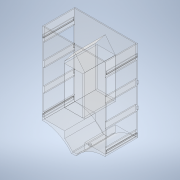
# Autodesk Inventor part: Contenedor
Saved by Autodesk Inventor 2021 (Build 250183000, 183)
## iProperties
Created: 2021-06-28
Part Number: Contenedor
Material: Acrílico, claro
Document SubType Name: Modeling
Designer: artur
Density: 1.19 g/cm^3
Appearance: Transparente - Claro
Mass: 3494.81 g
Surface Area: 8852.35 cm^2
Volume: 2936.81 cm^3
Author: artur
Autodesk Inventor part; units mm, degrees
ref_plane "YZ Plane" through (0, 0, 0) normal (1, 0, 0) x (0, 1, 0)
sketch "Boceto1" plane through (0, 0, 0) normal (0, 0, 1) x (1, 0, 0)
  line L0 (0, 0) -> (100, 0)
  line L1 (0, 300.0017) -> (0, 100.0017)
  line L2 (0, 0) -> (101, 0)
  line L3 (101, 0) -> (101, 400)
  line L4 (101, 400) -> (0, 400)
  line L5 (0, 300.0017) -> (0, 100.0017)
  line L6 (0, 0) -> (98.1777, 0) construction
  line L7 (98.1777, 0) -> (98.1777, 330) construction
  line L8 (98.1777, 330) -> (0, 330) construction
  line L9 (0, 330) -> (0, 0) construction
  line L10 (0, 300.0017) -> (-100, 300.0017) construction
  line L11 (-100, 300.0017) -> (-100, 100.0017) construction
  line L12 (-100, 100.0017) -> (0, 100.0017) construction
  line L13 (0, 100.0017) -> (0, 300.0017) construction
  line L14 (0, 300.0017) -> (-100, 300.0017)
  line L15 (-100, 300.0017) -> (-100, 100.0017)
  line L16 (-100, 100.0017) -> (0, 100.0017)
  line L17 (0, 100.0017) -> (0, 300.0017)
  line L18 (-100, 0) -> (-201, 0)
  line L19 (-201, 0) -> (-201, 400)
  line L20 (-201, 400) -> (-100, 400)
  line L21 (-100, 300.0017) -> (-100, 100.0017)
  line L22 (-100, 0) -> (0, 0)
  line L23 (-100, 400) -> (0, 400)
  line L24 (-95, 105.0017) -> (-5, 105.0017)
  line L25 (-5, 105.0017) -> (-5, 295.0017)
  line L26 (-5, 295.0017) -> (-95, 295.0017)
  line L27 (-95, 295.0017) -> (-95, 105.0017)
  line L28 (106, 400) -> (106, -5)
  line L29 (106, -5) -> (-206, -5)
  line L30 (-206, -5) -> (-206, 400)
  line L31 (-206, 400) -> (-201, 400)
  line L32 (101, 400) -> (106, 400)
  line L33 (-100, 100.0017) -> (-100, 0) construction
  line L34 (-50, -5) -> (-50, -75) construction
  line L35 (-56.35, -74.8888) -> (-43.65, -74.8888)
  line L36 (-43.65, -74.8888) -> (-38.65, -74.8888)
  line L37 (-56.35, -74.8888) -> (-61.35, -74.8888)
  arc A0 (-61.35, -74.8888) -> (-206, -5) centre (-206.1755, -189.9999) ccw
  arc A1 (106, -5) -> (-38.65, -74.8888) centre (106.1755, -189.9999) ccw
  line L38 (-38.65, -74.8888) -> (-38.65, -69.8888)
  line L39 (-61.35, -74.8888) -> (-61.35, -69.8888)
  arc A2 (-61.35, -69.8888) -> (-201, 0) centre (-206.2343, -184.9259) ccw
  arc A3 (98.1777, 0) -> (-38.65, -69.8888) centre (106.3177, -184.8208) ccw
  line L40 (-61.35, -69.8888) -> (-38.65, -69.8888)
  line L41 (-100, 0) -> (-100, -33.4687)
  line L42 (0, 0) -> (0, -33.4222)
  line L43 (-100, 400) -> (-100, 300.0017) construction
  dimension "d2" = 101
  dimension "d9" = 101
  dimension "d11" = 400
  dimension "d12" = 100
  dimension "d13" = 200
  dimension "d14" = 100
  dimension "d15" = 5
  dimension "d16" = 5
  dimension "d17" = 5
  dimension "d18" = 5
  dimension "d19" = 5
  dimension "d20" = 5
  dimension "d22" = 70
  dimension "d23" = 12.7
  dimension "d24" = 6.35
  dimension "d27" = 302
  dimension "d28" = 5
  dimension "d29" = 5
  dimension "d30" = 185
  dimension "d31" = 185
  dimension "d32" = 5
  dimension "d33" = 5
  dimension "d34" = 185
  dimension "d35" = 185
  dimension "d36" = 5
  constraints: 88 end point, 13 horizontal, 13 parallel, 10 point on circle, 8 perpendicular, 4 centre point, 4 vertical, 3 point on line, 2 collinear, 1 midpoint
  measures "d2" distance of L3.end L4.end
  measures "d9" distance of L19.end L20.end
  measures "d11" distance of L18.end L19.end
  measures "d12" distance of L20.end L4.end
  measures "d13" distance of L10.end L11.end
  measures "d14" distance of L11.end L1.end
  measures "d15" distance between parallel lines of L26 L10
  measures "d16" distance between parallel lines of L24 L12
  measures "d17" distance between parallel lines of L1 L25
  measures "d18" distance between parallel lines of L27 L11
  measures "d19" distance between parallel lines of L19 L30
  measures "d20" distance between parallel lines of L18 L29
  measures "d22" distance of L34.start L34.end
  measures "d23" distance of L35.start L35.end
  measures "d24" distance from line of L34 L35.end
  measures "d27" distance between parallel lines of L3 L19
  measures "d28" distance of L35.end L36.end
  measures "d29" distance of L35.start L37.end
  measures "d30" radius of A0
  measures "d31" radius of A1
  measures "d32" distance of L36.end L38.end
  measures "d33" distance of L37.end L39.end
  measures "d34" radius of A2
  measures "d35" radius of A3
  measures "d36" distance between parallel lines of L28 L3
extrude "Extrusión1" add sketch "Boceto1" against normal blind 152 contours L0 A3 L29 L42 | L0 L2 L3 L32 L28 L29 A3 | L41 L29 A2 L18 | L29 A3 L42 | L29 A1 L38 A3 | A2 L29 L30 L31 L19 | L41 A2 L29 | A2 L39 A0 L29 | L38 L36 L35 L37 L39 L40 | L1 L16 L15 L14
sketch "Boceto2" plane through (0, 0, 0) normal (0, 0, 1) x (1, 0, 0)
  line L0 (-206, 400) -> (-206, -5) projected
  line L1 (106, -5) -> (106, 400) projected
  arc A0 (106, -5) -> (-38.65, -74.8888) centre (106.1755, -189.9999) ccw projected
  arc A1 (-61.35, -74.8888) -> (-206, -5) centre (-206.1755, -189.9999) ccw projected
  line L2 (-61.35, -74.8888) -> (-38.65, -74.8888) projected
  line L3 (-206, 400) -> (106, 400)
  line L4 (-201, 0) -> (-201, 400) projected
  line L5 (0, 300.0017) -> (-100, 300.0017) projected
  line L6 (0, 100.0017) -> (0, 300.0017) projected
  line L7 (-95, 105.0017) -> (-95, 295.0017) projected
  line L8 (-5, 295.0017) -> (-5, 105.0017) projected
  line L9 (-5, 105.0017) -> (-95, 105.0017) projected
  line L10 (-95, 295.0017) -> (-5, 295.0017) projected
  point P0 (0, 0)
  constraints: 2 end point, 1 perpendicular
extrude "Extrusión2" add sketch "Boceto2" along normal blind 5
ref_plane "Plano de trabajo1" through (106, -5, -152) normal (0, 0, -1) x (-1, 0, 0)
sketch "Boceto5" plane through (106, -5, -152) normal (0, 0, -1) x (-1, 0, 0)
  line L0 (312, 0) -> (312, 405) projected
  line L1 (312, 405) -> (307, 405) projected
  line L2 (5, 405) -> (307, 405) projected
  line L3 (5, 405) -> (0, 405) projected
  line L4 (0, 405) -> (0, 0) projected
  arc A0 (144.65, -69.8888) -> (0, 0) centre (-0.1755, -184.9999) ccw projected
  line L5 (144.65, -69.8888) -> (167.35, -69.8888) projected
  arc A1 (312, 0) -> (167.35, -69.8888) centre (312.1755, -184.9999) ccw projected
  line L6 (201, 110.0017) -> (111, 110.0017) projected
  line L7 (111, 110.0017) -> (111, 300.0017) projected
  line L8 (111, 300.0017) -> (201, 300.0017) projected
  line L9 (201, 300.0017) -> (201, 110.0017) projected
  point P0 (106, 5)
extrude "Extrusión3" add sketch "Boceto5" along normal blind 5
sketch "Boceto6" plane through (-61.35, -74.8888, 5) normal (0, -1, 0) x (1, 0, 0)
  line L0 (-144.65, -162) -> (167.35, -162) construction
  line L1 (11.35, -162) -> (11.35, -25.687) construction
  line L2 (0, -5) -> (0, -157) construction
  line L3 (0, -81) -> (22.7, -81) construction
  line L4 (22.7, -5) -> (22.7, -157) construction
  circle A0 centre (11.35, -81) radius 6.35
  point P0 (61.35, -5)
  dimension "d76" = 12.7
  constraints: 4 end point, 4 midpoint, 1 centre point, 1 vertical
  measures "d76" diameter of A0
extrude "Extrusión4" cut sketch "Boceto6" against normal blind 5
sketch "Boceto7" plane through (-206, -5, 5) normal (-1, 0, 0) x (0, 0, 1)
  line L0 (-162, 0) -> (0, 0) construction
  line L1 (-81, 0) -> (-81, 5) construction
  line L2 (-81, 5) -> (-81, 35) construction
  line L3 (-81, 35) -> (-81, 115) construction
  line L4 (-81, 115) -> (-81, 145) construction
  line L5 (-81, 145) -> (-81, 225) construction
  line L6 (-81, 225) -> (-81, 255) construction
  line L7 (-81, 255) -> (-81, 335) construction
  line L8 (-157, 35) -> (-5, 35)
  line L9 (-5, 35) -> (-5, 115)
  line L10 (-5, 115) -> (-157, 115)
  line L11 (-157, 115) -> (-157, 35)
  line L12 (0, 405) -> (0, 0) projected
  line L13 (-162, 0) -> (-162, 405) projected
  line L14 (-5, 225) -> (-157, 225)
  line L15 (-157, 225) -> (-157, 145)
  line L16 (-157, 145) -> (-5, 145)
  line L17 (-5, 145) -> (-5, 225)
  line L18 (-5, 335) -> (-157, 335)
  line L19 (-157, 335) -> (-157, 255)
  line L20 (-157, 255) -> (-5, 255)
  line L21 (-5, 255) -> (-5, 335)
  point P0 (-5, 5)
  dimension "d47" = 5
  dimension "d48" = 30
  dimension "d49" = 80
  dimension "d50" = 30
  dimension "d51" = 80
  dimension "d52" = 30
  dimension "d53" = 80
  dimension "d54" = 5
  dimension "d55" = 5
  dimension "d58" = 110
  constraints: 38 end point, 6 point on line, 2 parallel, 2 vertical, 1 horizontal, 1 midpoint, 1 perpendicular, 16 other
  measures "d47" distance of L1.start L1.end
  measures "d48" distance of L1.end L2.end
  measures "d49" distance of L2.end L3.end
  measures "d50" distance of L3.end L4.end
  measures "d51" distance of L4.end L5.end
  measures "d52" distance of L5.end L6.end
  measures "d53" distance of L6.end L7.end
  measures "d54" distance between parallel lines of L12 L9
  measures "d55" distance between parallel lines of L13 L11
  measures "d58" distance of L9.end L14.start
sketch "Boceto8" plane through (106, -5, 5) normal (1, 0, 0) x (0, 0, -1)
  line L0 (5, 335) -> (157, 335) projected
  line L1 (157, 335) -> (157, 255) projected
  line L2 (157, 255) -> (5, 255) projected
  line L3 (5, 255) -> (5, 335) projected
  line L4 (5, 225) -> (157, 225) projected
  line L5 (157, 225) -> (157, 145) projected
  line L6 (157, 145) -> (5, 145) projected
  line L7 (5, 145) -> (5, 225) projected
  line L8 (5, 115) -> (157, 115) projected
  line L9 (157, 115) -> (157, 35) projected
  line L10 (157, 35) -> (5, 35) projected
  line L11 (5, 35) -> (5, 115) projected
  point P0 (5, 5)
extrude "Extrusión5" cut sketch "Boceto7" against normal blind 5
extrude "Extrusión6" cut sketch "Boceto8" against normal blind 5
sketch "Boceto9" plane through (106, -5, -152) normal (0, 0, 1) x (1, 0, 0)
  line L0 (0, 405) -> (0, 0) construction
  line L1 (0, 372.4568) -> (-312, 372.4568) construction
  line L2 (-312, 0) -> (-312, 405) construction
  line L3 (-156, 372.4568) -> (-156, 300.0017) construction
  line L4 (-111, 300.0017) -> (-201, 300.0017) construction
  line L5 (-312, 405) -> (0, 405) construction
  line L6 (-156, 405) -> (-156, 385) construction
  line L7 (-106, 405) -> (-106, 305) construction
  line L8 (-106, 305) -> (-206, 305) construction
  line L9 (-206, 305) -> (-106, 305)
  line L10 (-206, 305) -> (-156, 367.45)
  line L11 (-106, 305) -> (-156, 367.45)
  point P0 (-106, 5)
  dimension "d71" = 20
  dimension "d72" = 100
  dimension "d73" = 80
  constraints: 16 end point, 4 point on line, 3 midpoint, 2 vertical, 1 collinear, 1 horizontal, 1 perpendicular
  measures "d71" distance of L6.start L6.end
  measures "d72" distance of L7.start L7.end
  measures "d73" distance of L8.end L10.end
extrude "Extrusión7" add sketch "Boceto9" along normal blind 152
thread "Rosca1" size "M14x2" class "6H" standard "ANSI Metric M Profile" full length
sketch "Boceto11" plane through (106, -5, 5) normal (1, 0, 0) x (0, 0, -1)
  line L0 (157, 405) -> (157, 335) projected
  line L1 (5, 350) -> (157, 350)
  line L2 (157, 350) -> (157, 365)
  line L3 (157, 365) -> (5, 365)
  line L4 (5, 365) -> (5, 350)
  line L5 (5, 105.0017) -> (5, 305.0017) projected
  line L6 (5, 10) -> (157, 10)
  line L7 (157, 10) -> (157, 25)
  line L8 (157, 25) -> (5, 25)
  line L9 (5, 25) -> (5, 10)
  line L10 (162, 405) -> (0, 405) projected
  line L11 (157, 35) -> (5, 35) projected
  line L12 (0, 405) -> (0, 0) projected
  line L13 (5, 122.5) -> (0, 122.5)
  line L14 (0, 122.5) -> (0, 137.5)
  line L15 (0, 137.5) -> (5, 137.5)
  line L16 (5, 137.5) -> (5, 122.5)
  line L17 (5, 232.5) -> (0, 232.5)
  line L18 (0, 232.5) -> (0, 247.5)
  line L19 (0, 247.5) -> (5, 247.5)
  line L20 (5, 247.5) -> (5, 232.5)
  line L21 (157, 255) -> (5, 255) projected
  line L22 (5, 225) -> (157, 225) projected
  line L23 (157, 145) -> (5, 145) projected
  line L24 (5, 115) -> (157, 115) projected
  point P0 (5, 5)
  dimension "d79" = 152
  dimension "d80" = 40
  dimension "d81" = 15
  dimension "d84" = 15
  dimension "d89" = 10
  dimension "d92" = 7.5
  dimension "d93" = 7.5
  dimension "d94" = 7.5
  dimension "d95" = 7.5
  constraints: 32 end point, 8 parallel, 5 point on line, 4 horizontal, 4 perpendicular
  measures "d79" distance of L2.end L3.end
  measures "d80" distance between parallel lines of L10 L3
  measures "d81" distance between parallel lines of L1 L3
  measures "d84" distance of L8.end L6.start
  measures "d89" distance between parallel lines of L11 L8
  measures "d92" distance between parallel lines of L21 L19
  measures "d93" distance between parallel lines of L17 L22
  measures "d94" distance between parallel lines of L23 L15
  measures "d95" distance between parallel lines of L13 L24
extrude "Extrusión8" add sketch "Boceto11" along normal blind 3 contours L0 L1 L4 L3 | L19 L5 L17 L12 | L15 L5 L13 L12 | L9 L8 L7 L6
sketch "Boceto12" plane through (106, 345, -152) normal (0, -1, 0) x (1, 0, 0)
  line L0 (1, 152) -> (2, 152)
  line L1 (2, 152) -> (2, 0)
  line L2 (2, 0) -> (1, 0)
  line L3 (1, 0) -> (1, 152)
  line L4 (0, 152) -> (0, 0) projected
  line L5 (0, 152) -> (3, 152) projected
  line L6 (0, 0) -> (3, 0) projected
  point P0 (-106, 152)
  dimension "d96" = 1
  dimension "d97" = 1
  dimension "d98" = 0
  dimension "d99" = 0
  constraints: 8 end point, 2 parallel, 1 horizontal, 1 perpendicular
  measures "d96" distance between parallel lines of L3 L4
  measures "d97" distance between parallel lines of L1 L3
  measures "d98" distance between parallel lines of L5 L0
  measures "d99" distance between parallel lines of L6 L2
extrude "Extrusión9" cut sketch "Boceto12" against normal blind 5 contours L0 L1 L2 L3
sketch "Boceto13" plane through (106, 20, 0) normal (0, 1, 0) x (1, 0, 0)
  line L0 (2, 0) -> (1, 0)
  line L1 (1, 0) -> (1, 152)
  line L2 (1, 152) -> (2, 152)
  line L3 (2, 152) -> (2, 0)
  line L4 (0, 0) -> (3, 0) projected
  line L5 (0, 0) -> (0, 152) projected
  line L6 (0, 152) -> (3, 152) projected
  point P0 (-106, 0)
  dimension "d102" = 0
  dimension "d103" = 1
  dimension "d104" = 1
  dimension "d105" = 0
  constraints: 8 end point, 2 parallel, 1 horizontal, 1 perpendicular
  measures "d102" distance between parallel lines of L4 L0
  measures "d103" distance between parallel lines of L1 L3
  measures "d104" distance between parallel lines of L1 L5
  measures "d105" distance between parallel lines of L6 L2
extrude "Extrusión10" cut sketch "Boceto13" against normal blind 5 contours L0 L1 L2 L3
ref_plane "Plano de trabajo2" through (-50, -5, -157) normal (1, 0, 0) x (0, 0, -1)
mirror "Simetría1" about plane through (-50, -5, -157) normal (1, 0, 0) of "Extrusión8"
sketch "Boceto14" plane through (-206, 20, 0) normal (0, 1, 0) x (1, 0, 0)
  line L0 (-2, 152) -> (-1, 152)
  line L1 (-1, 152) -> (-1, 0)
  line L2 (-1, 0) -> (-2, 0)
  line L3 (-2, 0) -> (-2, 152)
  line L4 (0, 152) -> (-3, 152) projected
  line L5 (-3, 152) -> (-3, 0) projected
  line L6 (0, 0) -> (-3, 0) projected
  point P0 (206, 0)
  dimension "d108" = 0
  dimension "d109" = 1
  dimension "d110" = 1
  dimension "d111" = 0
  constraints: 8 end point, 2 parallel, 1 horizontal, 1 perpendicular
  measures "d108" distance between parallel lines of L4 L0
  measures "d109" distance between parallel lines of L5 L3
  measures "d110" distance between parallel lines of L1 L3
  measures "d111" distance between parallel lines of L6 L2
extrude "Extrusión11" cut sketch "Boceto14" against normal blind 5 contours L0 L1 L2 L3
sketch "Boceto15" plane through (-206, 345, -152) normal (0, -1, 0) x (1, 0, 0)
  line L0 (-1, 0) -> (-2, 0)
  line L1 (-2, 0) -> (-2, 152)
  line L2 (-2, 152) -> (-1, 152)
  line L3 (-1, 152) -> (-1, 0)
  line L4 (0, 0) -> (-3, 0) projected
  line L5 (-3, 0) -> (-3, 152) projected
  line L6 (0, 152) -> (-3, 152) projected
  point P0 (206, 152)
  dimension "d114" = 0
  dimension "d115" = 1
  dimension "d116" = 1
  dimension "d117" = 0
  constraints: 8 end point, 2 parallel, 1 horizontal, 1 perpendicular
  measures "d114" distance between parallel lines of L4 L0
  measures "d115" distance between parallel lines of L5 L1
  measures "d116" distance between parallel lines of L1 L3
  measures "d117" distance between parallel lines of L6 L2
extrude "Extrusión12" cut sketch "Boceto15" against normal blind 5 contours L0 L1 L2 L3
equation "\"d16\" = d15"
equation "\"d17\" = d15"
equation "\"d18\" = d15"
equation "\"d19\" = d15"
equation "\"d20\" = d15"
equation "\"d24\" = 0.5 * d23"
equation "\"d31\" = d30"
equation "\"d84\" = d81"
